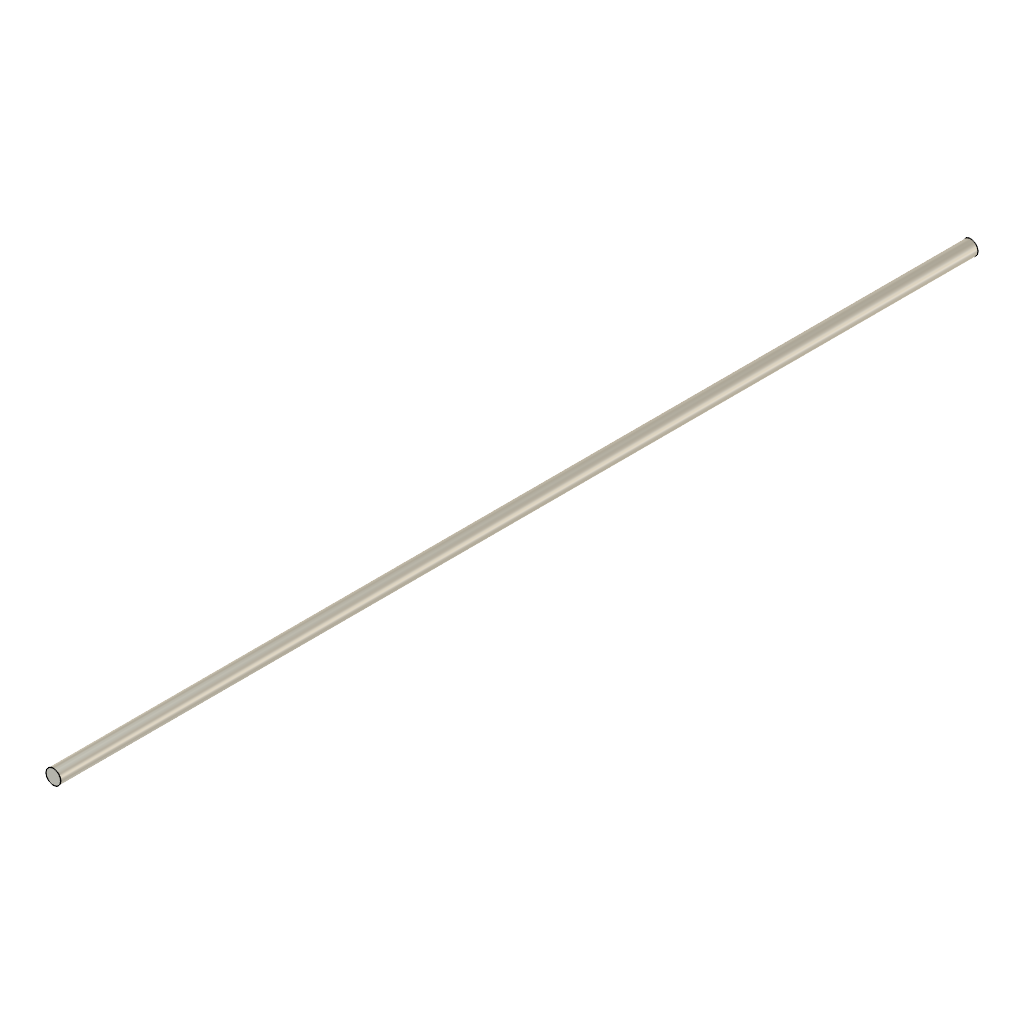
FEA_BEAM (Autodesk Fusion 360 design; units mm, degrees)
part number: 2026-09-09-23-34-09-178
Autodesk Fusion 360 part; units mm, degrees
sketch "Sketch3" plane through (0, 0, 0) normal (0, 1, 0) x (1, 0, 0)
  circle A0 centre (0, 0) radius 4.445
  dimension "d13" = 8.89
  constraint coincident A0.centre origin
  measures "d13" diameter of A0
extrude "Extrude3" add sketch "Sketch3" along normal blind 549.91
equation "Diameter = 0.75 in"
equation "Delta = 0.009 in"
equation "Force = ( 400 lbforce ) / lbforce"
equation "Elastic_Modulus = ( 10000000 ksi ) / ksi"
equation "Area = PI * pow(Diameter / 2 in; 2)"
equation "Length = ( Delta * Area * Elastic_Modulus ) / Force"
